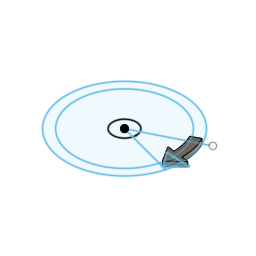
2023_03_04_Rotation Arrows Axis v5 (Autodesk Fusion 360 design; units mm, degrees)
Autodesk Fusion 360 part; units mm, degrees
note: some values were not read from the file. Set by a fixed rule: which sketch regions a step uses.
sketch "Sketch1" plane through (0, 0, 0) normal (0, 0, 1) x (1, 0, 0)
  circle A0 centre (0, 0) radius 5
  circle A1 centre (0, 0) radius 25
  circle A2 centre (0, 0) radius 21
  line L0 (21, 0) -> (25, 0)
  line L1 (23, 0) -> (28, 0)
  line L2 (23, 0) -> (18, 0)
  line L3 (18, 0) -> (23, 0)
  line L4 (23, -6) -> (28, 0)
  line L5 (23, -6) -> (18, 0)
  line L6 (0, 0) -> (25.5, 12.5676)
  line L7 (0, 0) -> (24.156, -6.441)
  line L8 (20.2911, -5.4105) -> (24.156, -6.441)
  line L9 (22.2235, -5.9257) -> (23, 0)
  line L10 (23, 0) -> (18.0424, 0.6496)
  line L11 (23, 0) -> (27.9576, -0.6496)
  line L12 (27.9576, -0.6496) -> (22.2235, -5.9257)
  line L13 (22.2235, -5.9257) -> (18.0424, 0.6496)
  dimension "d1" = 10
  dimension "d4" = 90
  dimension "d5" = 5
  dimension "d6" = 5
  constraint coincident A0.centre A1.centre
  constraint concentric A1 A2
  constraint coincident A2 L0.start
  constraint coincident A1 L0.end
  constraint horizontal L0
  constraint midpoint L0 L1.start
  constraint parallel L0 L1
  constraint parallel L0 L2
  constraint coincident A1 L7.end
  constraint coincident A2 L8.start
  constraint coincident L7 L8.start
  constraint midpoint L8 L9.start
  constraint perpendicular L9 L11
  measures "d1" diameter of A0
  measures "d4" angle of L9 L10
  measures "d5" distance of L1.start L10.end
  measures "d6" distance of L1.start L11.end
extrude "Extrude1" add sketch "Sketch1" along normal blind 2 contours A1 A2 L0 L1 L6 L10 | A2 L0 L2 L3 L10 | A2 L0 L2 L3 L5 L9 | A2 L2 L3 L5 L13 | A1 L5 L9 L11 L12 | A1 L0 L1 L11 | A1 L1 L4 L11 | L2 L3 L5 L13 | A1 L4 L5 L12 | A1 L4 L11 L12 | A1 L4 L12 makes body 1
move_body "Move1" bodies 1 to x (1, 0, 0) y (0, 1, 0) z (0, 0, 1) at (14, 0, 0)
extrude "Extrude2" add sketch "Sketch1" along normal blind 2 separate body contours A1 A2 L0 L1 L6 L10 | A2 L0 L2 L3 L10 | A2 L2 L3 L10 L13 | A2 L5 L13 | A2 L5 L9 L13 | L5 L9 L12 | A2 L0 L2 L3 L5 L9 | A2 L2 L3 L5 L13 | A1 L5 L9 L11 L12 | A1 L0 L1 L11 | A1 L4 L11 L12 | L4 L11 L12 makes body 2
hidden bodies 1
